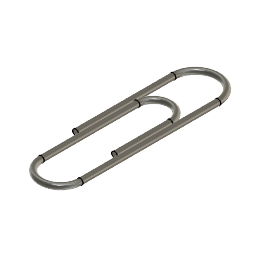
Paperclip (Autodesk Fusion 360 design; units mm, degrees)
part number: 2026-02-10-12-05-16-528
Autodesk Fusion 360 part; units mm, degrees
sketch "Sketch1" plane through (0, 0, 0) normal (0, 0, 1) x (1, 0, 0)
  line L0 (0, 0) -> (0, 16.25)
  line L1 (7.5, 16.25) -> (7.5, -6.75)
  line L2 (1, -6.75) -> (1, 9.25)
  line L3 (6.5, 9.25) -> (6.5, 0)
  arc A0 (3.75, 20) -> (0, 16.25) centre (3.75, 16.25) ccw
  arc A1 (7.5, 16.25) -> (3.75, 20) centre (3.75, 16.25) ccw
  arc A2 (1, -6.75) -> (4.25, -10) centre (4.25, -6.75) ccw
  arc A3 (4.25, -10) -> (7.5, -6.75) centre (4.25, -6.75) ccw
  arc A4 (3.75, 12) -> (1, 9.25) centre (3.75, 9.25) ccw
  arc A5 (6.5, 9.25) -> (3.75, 12) centre (3.75, 9.25) ccw
  point P0 (0, 20)
  point P1 (7.5, 20)
  point P2 (7.5, -10)
  point P3 (1, -10)
  point P4 (1, 12)
  point P5 (6.5, 12)
  dimension "d2" = 20
  dimension "d4" = 7.5
  dimension "d6" = 30
  dimension "d8" = 6.5
  dimension "d10" = 22
  dimension "d12" = 5.5
  dimension "d14" = 12
  dimension "d15" = 3.75
  dimension "d16" = 3.75
  dimension "d17" = 3.25
  dimension "d18" = 3.25
  dimension "d19" = 2.75
  dimension "d20" = 2.75
  constraint vertical L0
  constraint coincident L0.start origin
  constraint coincident P0 L0
  constraint tangent L0 A0
  constraint coincident P1 L1
  constraint tangent L1 A1
  constraint coincident A0.start A1.end
  constraint coincident P3 L2
  constraint tangent L2 A2
  constraint coincident P2 L1
  constraint tangent L1 A3
  constraint coincident A2.end A3.start
  constraint coincident P4 L2
  constraint tangent L2 A4
  constraint coincident P5 L3
  constraint tangent L3 A5
  constraint coincident A4.start A5.end
  measures "d2" distance of L0.start P0
  measures "d4" distance of P0 P1
  measures "d6" distance of P1 P2
  measures "d8" distance of P2 P3
  measures "d10" distance of P3 P4
  measures "d12" distance of P4 P5
  measures "d14" distance of P5 L3.end
  measures "d15" radius of A0
  measures "d16" radius of A1
  measures "d17" radius of A2
  measures "d18" radius of A3
  measures "d19" radius of A4
  measures "d20" radius of A5
sketch "Sketch2" plane through (0, 0, 0) normal (0, 1, 0) x (1, 0, 0)
  circle A0 centre (0, 0) radius 0.5
  dimension "d21" = 1
  constraint coincident A0.centre origin
  measures "d21" diameter of A0
sweep "Sweep1" add profiles "Sketch2" path "Sketch1" along L0 A0 A1 L1 A3 A2 L2 A4 A5 L3 section 1
